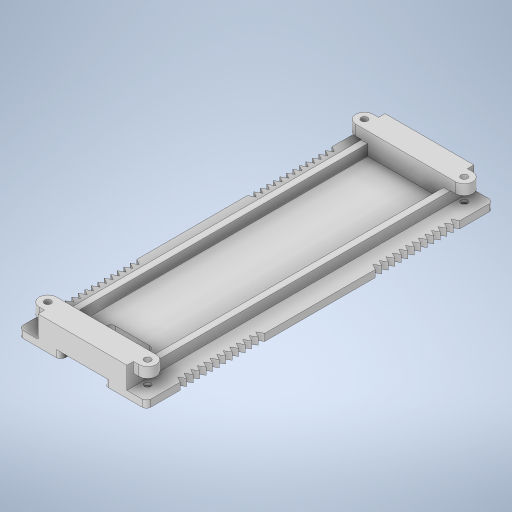
# Autodesk Inventor part: BatteryCarrier SlideRail ToothMountPlate
Saved by Autodesk Inventor 2023 (Build 270158000, 158)
## iProperties
Created: 2023-01-18
Part Number: BatteryCarrier SlideRail ToothMountPlate
Material: Generic
Document SubType Name: Modeling
Designer: Administrator
Density: 1 g/cm^3
Appearance: Default
Author: Administrator
Autodesk Inventor part; units mm, degrees
ref_plane "YZ Plane" through (0, 0, 0) normal (1, 0, 0) x (0, 1, 0)
ref_plane "XZ Plane" through (0, 0, 0) normal (0, 1, 0) x (-1, 0, 0)
ref_plane "XY Plane" through (0, 0, 0) normal (0, 0, 1) x (1, 0, 0)
sketch "Sketch1" plane through (0, 0, 0) normal (0, 0, 1) x (1, 0, 0)
  line L0 (0, 0) -> (146, 0) construction
  line L1 (146, 0) -> (146, 46) construction
  line L2 (146, 46) -> (0, 46) construction
  line L3 (0, 46) -> (0, 0) construction
  circle A0 centre (0, 46) radius 1.5
  circle A1 centre (0, 0) radius 1.5
  circle A2 centre (146, 0) radius 1.5
  circle A3 centre (146, 46) radius 1.5
  line L4 (0, 0) -> (146, 46) construction
  line L5 (-7, -6.5) -> (153, -6.5)
  line L6 (153, -6.5) -> (153, 52.5)
  line L7 (153, 52.5) -> (-7, 52.5)
  line L8 (-7, 52.5) -> (-7, -6.5)
  line L9 (-7, -6.5) -> (153, 52.5) construction
  line L10 (153, -6.5) -> (-7, 52.5) construction
  line L11 (73, 23) -> (93, 23) construction
  line L12 (73, 23) -> (73, 43) construction
  line L13 (116.5, -6.5) -> (118, -3.9019)
  line L14 (116.5, -6.5) -> (119.5, -6.5) construction
  line L15 (118, -3.9019) -> (119.5, -6.5)
  line L16 (26.5, -6.5) -> (28, -3.9019)
  line L17 (26.5, -6.5) -> (29.5, -6.5) construction
  line L18 (28, -3.9019) -> (29.5, -6.5)
  line L19 (26.5, -6.5) -> (29.5, -6.5)
  line L20 (119.5, -6.5) -> (116.5, -6.5)
  line L21 (-7, 33) -> (16, 33)
  line L22 (16, 33) -> (16, 13)
  line L23 (16, 13) -> (-7, 13)
  line L24 (-7, 13) -> (-7, 33)
  dimension "d0" = 146
  dimension "d1" = 46
  dimension "d2" = 3
  dimension "d3" = 3
  dimension "d4" = 3
  dimension "d5" = 3
  dimension "d6" = 160
  dimension "d7" = 59
  dimension "d8" = 20
  dimension "d9" = 20
  dimension "d10" = 3
  dimension "d11" = 60
  dimension "d12" = 3
  dimension "d13" = 60
  dimension "d14" = 3
  dimension "d15" = 60
  dimension "d16" = 3
  dimension "d17" = 60
  dimension "d18" = 90
  dimension "d19" = 35
  dimension "d30" = 23
  dimension "d31" = 20
  dimension "d32" = 19.5
  constraints: 50 end point, 6 horizontal, 6 parallel, 4 centre point, 4 coincident, 4 perpendicular, 3 midpoint, 2 collinear, 2 equal length, 1 point on line
  measures "d0" distance of L2.end L1.end
  measures "d1" distance of L1.end L0.end
  measures "d2" diameter of A0
  measures "d3" diameter of A1
  measures "d4" diameter of A2
  measures "d5" diameter of A3
  measures "d6" distance of L7.end L6.end
  measures "d7" distance of L6.end L5.end
  measures "d8" distance of L11.start L11.end
  measures "d9" distance of L11.start L12.end
  measures "d10" distance of L13.start L13.end
  measures "d11" angle of L14 L13
  measures "d12" distance of L13.end L15.end
  measures "d13" angle of L13 L15
  measures "d14" distance of L16.start L16.end
  measures "d15" angle of L17 L16
  measures "d16" distance of L16.end L18.end
  measures "d17" angle of L16 L18
  measures "d18" distance of L13.end L16.end
  measures "d19" distance from line of L6 L13.end
  measures "d30" distance of L22.end L23.end
  measures "d31" distance of L21.end L22.end
  measures "d32" distance between parallel lines of L7 L21
extrude "Extrusion1" add sketch "Sketch1" along normal blind 3.25 contours L8 L23 L22 L21 L7 L6 L5 L15 L13 L18 L16
extrude "Extrusion2" cut sketch "Sketch1" along normal blind 10 contours L16 L18 L5 | L13 L15 L5
pattern_linear "Rectangular Pattern1" count 7 spacing 3 along (1, 0, 0) of "Extrusion2"
pattern_linear "Rectangular Pattern2" count 7 spacing 3 along (-1, 0, 0) of "Extrusion2"
ref_plane "Work Plane1" through (-7, 23, 0) normal (0, 1, 0) x (1, 0, 0)
mirror "Mirror1" about plane through (-7, 23, 0) normal (0, 1, 0) of "Extrusion2", "Rectangular Pattern1", "Rectangular Pattern2"
fillet "Fillet1" radius 2 8 edges at (-7, 52.5, 1.625) (-7, 13, 1.625) (-7, -6.5, 1.625) (-7, 33, 1.625) (153, 52.5, 1.625) (153, -6.5, 1.625) (16, 13, 1.625) (16, 33, 1.625)
chamfer "Chamfer1" distance 2 angle 45 4 edges at (-1.5, 46, 3.25) (-1.5, 0, 3.25) (144.5, 46, 3.25) (144.5, 0, 3.25)
sketch "Sketch3" plane through (0, 0, 0) normal (0, 0, -1) x (-1, 0, 0)
  circle A0 centre (-146, 46) radius 1.5 construction
  circle A1 centre (0, 0) radius 1.5 construction
  line L0 (-146, 46) -> (0, 46) construction
  line L1 (0, 46) -> (0, 0) construction
  line L2 (0, 0) -> (-146, 0) construction
  line L3 (-146, 0) -> (-146, 46) construction
  line L4 (-153, 43.5) -> (-142, 43.5)
  line L5 (-142, 43.5) -> (-142, 2.5)
  line L6 (-142, 2.5) -> (-153, 2.5)
  line L7 (-153, 2.5) -> (-153, 43.5)
  line L8 (7, 43.5) -> (-4, 43.5)
  line L9 (-4, 43.5) -> (-4, 2.5)
  line L10 (-4, 2.5) -> (7, 2.5)
  line L11 (7, 2.5) -> (7, 43.5)
  line L12 (-4, 43.5) -> (-142, 43.5)
  line L13 (-142, 43.5) -> (-142, 40.5)
  line L14 (-142, 40.5) -> (-4, 40.5)
  line L15 (-4, 40.5) -> (-4, 43.5)
  line L16 (-142, 2.5) -> (-4, 2.5)
  line L17 (-4, 2.5) -> (-4, 5.5)
  line L18 (-4, 5.5) -> (-142, 5.5)
  line L19 (-142, 5.5) -> (-142, 2.5)
  point P0 (-4, 40.5)
  point P1 (-4, 2.5)
  dimension "d46" = 2.5
  dimension "d47" = 2.5
  dimension "d48" = 7
  dimension "d50" = 4
  dimension "d51" = 7
  dimension "d52" = 4
  dimension "d63" = 3
  dimension "d64" = 3
  constraints: 40 end point, 10 parallel, 5 horizontal, 5 perpendicular, 2 point on line
  measures "d46" distance between parallel lines of L0 L4
  measures "d47" distance between parallel lines of L2 L6
  measures "d48" distance between parallel lines of L3 L7
  measures "d50" distance between parallel lines of L3 L5
  measures "d51" distance between parallel lines of L1 L11
  measures "d52" distance between parallel lines of L1 L9
  measures "d63" distance of L13.end L12.end
  measures "d64" distance of L17.end L16.end
extrude "Extrusion4" add sketch "Sketch3" along normal blind 10 contours L4 L5 L6 L7 | L8 L11 L10 L9
sketch "Sketch4" plane through (0, 0, -10) normal (0, 0, -1) x (-1, 0, 0)
  circle A0 centre (-146, 0) radius 1.5 projected
  circle A1 centre (-146, 46) radius 1.5 projected
  line L0 (-146, 0) -> (-146, 46) construction
  line L1 (-142, 0) -> (-142, 46)
  line L2 (-150, 46) -> (-150, 0)
  arc A2 (-150, 0) -> (-142, 0) centre (-146, 0) ccw
  arc A3 (-142, 46) -> (-150, 46) centre (-146, 46) ccw
  circle A4 centre (0, 0) radius 1.5 projected
  circle A5 centre (0, 46) radius 1.5 projected
  line L3 (0, 0) -> (0, 46) construction
  line L4 (4, 0) -> (4, 46)
  line L5 (-4, 46) -> (-4, 0)
  arc A6 (-4, 0) -> (4, 0) centre (0, 0) ccw
  arc A7 (4, 46) -> (-4, 46) centre (0, 46) ccw
  point P0 (-146, 23)
  point P1 (0, 23)
  constraints: 16 end point, 8 point on circle, 8 tangent, 4 centre point, 3 parallel, 2 midpoint
extrude "Extrusion5" add sketch "Sketch4" against normal blind 4.75
extrude "Extrusion6" add sketch "Sketch3" along normal blind 5 contours L12 L9 L14 L5 | L5 L18 L9 L16
equation "\"d19\" = -0.5 * d18 + 0.5 * d6"
equation "\"d32\" = -0.5 * d31 + 0.5 * d7"
body "Solid1"
